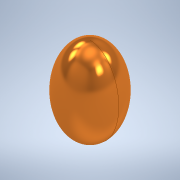
# Autodesk Inventor part: Ei_groß
Saved by Autodesk Inventor 2020 (Build 240168000, 168)
## iProperties
Created: 2021-05-12
Part Number: Ei_groß
Material: Gold
Document SubType Name: Modeling
Designer: Julian Uhl
Density: 19.3 g/cm^3
Appearance: Metall - 1600F (heiß)
Author: Julian Uhl
Autodesk Inventor part; units mm, degrees
ref_plane "YZ Plane" through (0, 0, 0) normal (1, 0, 0) x (0, 1, 0)
ref_plane "XZ Plane" through (0, 0, 0) normal (0, 1, 0) x (-1, 0, 0)
ref_plane "XY Plane" through (0, 0, 0) normal (0, 0, 1) x (1, 0, 0)
sketch "Skizze1" plane through (0, 0, 0) normal (0, 0, 1) x (1, 0, 0)
  line L0 (-42, 0) -> (42, 0) projected
  line L1 (0, -63) -> (0, 63) projected
  ellipse E0 centre (0, 0) end of major axis (-30, 0) minor radius 45
  point P0 (0, 45)
  point P1 (0, -45)
  dimension "d0" = 30
  dimension "d1" = 45
  constraints: 1 coincident, 2 other
revolve "Umdrehung1" add sketch "Skizze1" angle 360 about axis through (0, -10, 0) along (0, 1, 0) picked at (4.3803, 28.4844) picked at (3.0256, -29.297) contours L1 E0 L0 | L0 E0 L1
